Autodesk Fusion 360 part; units mm, degrees
note: some values were not read from the file. Set by a fixed rule: which sketch regions a step uses.
(part 4 of 20)
  spline S18 degree 5 poles (-22.7084, -21.1029) (-22.7059, -21.1018) (-22.7009, -21.0998) (-22.6934, -21.0967) (-22.6834, -21.0925) (-22.671, -21.0873) (-22.6586, -21.0822) (-22.6462, -21.077) (-22.6339, -21.0718) (-22.6217, -21.0666) (-22.6094, -21.0614) (-22.5972, -21.0562) (-22.585, -21.051) (-22.5729, -21.0458) (-22.5608, -21.0406) (-22.5487, -21.0354) (-22.5367, -21.0302) (-22.5247, -21.025) (-22.5127, -21.0198) (-22.5008, -21.0145) (-22.4889, -21.0093) (-22.4771, -21.0041) (-22.4653, -20.9989) (-22.4535, -20.9937) (-22.4417, -20.9884) (-22.43, -20.9832) (-22.4184, -20.978) (-22.4067, -20.9727) (-22.3951, -20.9675) (-22.3836, -20.9623) (-22.3721, -20.957) (-22.3606, -20.9518) (-22.3491, -20.9466) (-22.3377, -20.9413) (-22.3264, -20.9361) (-22.315, -20.9308) (-22.3037, -20.9256) (-22.2925, -20.9204) (-22.2812, -20.9151) (-22.2701, -20.9099) (-22.2589, -20.9046) (-22.2478, -20.8994) (-22.2367, -20.8942) (-22.2257, -20.8889) (-22.2147, -20.8837) (-22.2038, -20.8784) (-22.1928, -20.8732) (-22.182, -20.868) (-22.1711, -20.8627) (-22.1603, -20.8575) (-22.1496, -20.8523) (-22.1388, -20.847) (-22.1281, -20.8418) (-22.1175, -20.8366) (-22.1069, -20.8313) (-22.0963, -20.8261) (-22.0858, -20.8209) (-22.0753, -20.8157) (-22.0649, -20.8105) (-22.0544, -20.8052) (-22.0441, -20.8) (-22.0337, -20.7948) (-22.0235, -20.7896) (-22.0132, -20.7844) (-22.003, -20.7792) (-21.9928, -20.774) (-21.9827, -20.7688) (-21.9726, -20.7636) (-21.9625, -20.7584) (-21.9525, -20.7532) (-21.9426, -20.748) (-21.9326, -20.7429) (-21.9228, -20.7377) (-21.9129, -20.7325) (-21.9031, -20.7274) (-21.8933, -20.7222) (-21.8836, -20.717) (-21.8739, -20.7119) (-21.8643, -20.7067) (-21.8547, -20.7016) (-21.8451, -20.6965) (-21.8356, -20.6913) (-21.8261, -20.6862) (-21.8167, -20.6811) (-21.8073, -20.676) (-21.798, -20.6709) (-21.7887, -20.6658) (-21.7794, -20.6607) (-21.7702, -20.6556) (-21.761, -20.6505) (-21.7519, -20.6454) (-21.7428, -20.6404) (-21.7337, -20.6353) (-21.7247, -20.6303) (-21.7158, -20.6252) (-21.7068, -20.6202) (-21.698, -20.6152) (-21.6891, -20.6101) (-21.6803, -20.6051) (-21.6716, -20.6001) (-21.6629, -20.5951) (-21.6542, -20.5902) (-21.6456, -20.5852) (-21.6371, -20.5802) (-21.6285, -20.5753) (-21.6201, -20.5703) (-21.6116, -20.5654) (-21.6032, -20.5605) (-21.5949, -20.5555) (-21.5866, -20.5506) (-21.5783, -20.5457) (-21.5701, -20.5409) (-21.5619, -20.536) (-21.5538, -20.5311) (-21.5458, -20.5263) (-21.5377, -20.5214) (-21.5297, -20.5166) (-21.5218, -20.5118) (-21.5139, -20.507) (-21.5061, -20.5022) (-21.4983, -20.4974) (-21.4905, -20.4927) (-21.4828, -20.4879) (-21.4752, -20.4832) (-21.4676, -20.4784) (-21.46, -20.4737) (-21.4525, -20.469) (-21.445, -20.4644) (-21.4376, -20.4597) (-21.4302, -20.455) (-21.4229, -20.4504) (-21.4156, -20.4458) (-21.4084, -20.4412) (-21.4012, -20.4366) (-21.3941, -20.432) (-21.387, -20.4274) (-21.38, -20.4229) (-21.373, -20.4184) (-21.3661, -20.4139) (-21.3592, -20.4094) (-21.3523, -20.4049) (-21.3455, -20.4004) (-21.3388, -20.396) (-21.3321, -20.3916) (-21.3255, -20.3872) (-21.3189, -20.3828) (-21.3124, -20.3784) (-21.3059, -20.3741) (-21.2995, -20.3698) (-21.2931, -20.3655) (-21.2867, -20.3612) (-21.2805, -20.3569) (-21.2742, -20.3527) (-21.2681, -20.3484) (-21.2619, -20.3442) (-21.2559, -20.3401) (-21.2498, -20.3359) (-21.2439, -20.3318) (-21.238, -20.3277) (-21.2321, -20.3236) (-21.2263, -20.3195) (-21.2205, -20.3155) (-21.2148, -20.3115) (-21.2092, -20.3075) (-21.2036, -20.3035) (-21.1981, -20.2996) (-21.1926, -20.2956) (-21.1871, -20.2918) (-21.1818, -20.2879) (-21.1764, -20.2841) (-21.1712, -20.2802) (-21.166, -20.2765) (-21.1608, -20.2727) (-21.1557, -20.269) (-21.1507, -20.2653) (-21.1457, -20.2616) (-21.1408, -20.258) (-21.1359, -20.2544) (-21.1311, -20.2508) (-21.1263, -20.2472) (-21.1216, -20.2437) (-21.117, -20.2402) (-21.1124, -20.2368) (-21.1079, -20.2333) (-21.1034, -20.23) (-21.099, -20.2266) (-21.0947, -20.2233) (-21.0904, -20.22) (-21.0862, -20.2167) (-21.082, -20.2135) (-21.0779, -20.2103) (-21.0739, -20.2072) (-21.0699, -20.2041) (-21.066, -20.201) (-21.0621, -20.198) (-21.0583, -20.195) (-21.0546, -20.192) (-21.0509, -20.1891) (-21.0473, -20.1862) (-21.0437, -20.1834) (-21.0403, -20.1806) (-21.0368, -20.1778) (-21.0335, -20.1751) (-21.0302, -20.1724) (-21.027, -20.1698) (-21.0238, -20.1672) (-21.0207, -20.1647) (-21.0177, -20.1622) (-21.0148, -20.1597) (-21.0119, -20.1573) (-21.009, -20.155) (-21.0063, -20.1527) (-21.0036, -20.1504) (-21.001, -20.1482) (-20.9984, -20.1461) (-20.996, -20.144) (-20.9936, -20.1419) (-20.9912, -20.1399) (-20.989, -20.138) (-20.9868, -20.1361) (-20.9847, -20.1343) (-20.9826, -20.1325) (-20.9806, -20.1308) (-20.9787, -20.1291) (-20.9769, -20.1275) (-20.9752, -20.126) (-20.9735, -20.1245) (-20.9719, -20.123) (-20.9704, -20.1217) (-20.9689, -20.1204) (-20.9675, -20.1192) (-20.9663, -20.118) (-20.9651, -20.1169) (-20.9639, -20.1159) (-20.9629, -20.1149) (-20.9619, -20.114) (-20.961, -20.1132) (-20.9602, -20.1125) (-20.9595, -20.1118) (-20.9589, -20.1112) (-20.9583, -20.1107) (-20.958, -20.1104) (-20.9577, -20.1102) (-20.9576, -20.11) (-20.9575, -20.11) knots -1 -1 -1 -1 -1 -1 -0.99583333 -0.99166667 -0.9875 -0.98333333 -0.97916667 -0.975 -0.97083333 -0.96666667 -0.9625 -0.95833333 -0.95416667 -0.95 -0.94583333 -0.94166667 -0.9375 -0.93333333 -0.92916667 -0.925 -0.92083333 -0.91666667 -0.9125 -0.90833333 -0.90416667 -0.9 -0.89583333 -0.89166667 -0.8875 -0.88333333 -0.87916667 -0.875 -0.87083333 -0.86666667 -0.8625 -0.85833333 -0.85416667 -0.85 -0.84583333 -0.84166667 -0.8375 -0.83333333 -0.82916667 -0.825 -0.82083333 -0.81666667 -0.8125 -0.80833333 -0.80416667 -0.8 -0.79583333 -0.79166667 -0.7875 -0.78333333 -0.77916667 -0.775 -0.77083333 -0.76666667 -0.7625 -0.75833333 -0.75416667 -0.75 -0.74583333 -0.74166667 -0.7375 -0.73333333 -0.72916667 -0.725 -0.72083333 -0.71666667 -0.7125 -0.70833333 -0.70416667 -0.7 -0.69583333 -0.69166667 -0.6875 -0.68333333 -0.67916667 -0.675 -0.67083333 -0.66666667 -0.6625 -0.65833333 -0.65416667 -0.65 -0.64583333 -0.64166667 -0.6375 -0.63333333 -0.62916667 -0.625 -0.62083333 -0.61666667 -0.6125 -0.60833333 -0.60416667 -0.6 -0.59583333 -0.59166667 -0.5875 -0.58333333 -0.57916667 -0.575 -0.57083333 -0.56666667 -0.5625 -0.55833333 -0.55416667 -0.55 -0.54583333 -0.54166667 -0.5375 -0.53333333 -0.52916667 -0.525 -0.52083333 -0.51666667 -0.5125 -0.50833333 -0.50416667 -0.5 -0.49583333 -0.49166667 -0.4875 -0.48333333 -0.47916667 -0.475 -0.47083333 -0.46666667 -0.4625 -0.45833333 -0.45416667 -0.45 -0.44583333 -0.44166667 -0.4375 -0.43333333 -0.42916667 -0.425 -0.42083333 -0.41666667 -0.4125 -0.40833333 -0.40416667 -0.4 -0.39583333 -0.39166667 -0.3875 -0.38333333 -0.37916667 -0.375 -0.37083333 -0.36666667 -0.3625 -0.35833333 -0.35416667 -0.35 -0.34583333 -0.34166667 -0.3375 -0.33333333 -0.32916667 -0.325 -0.32083333 -0.31666667 -0.3125 -0.30833333 -0.30416667 -0.3 -0.29583333 -0.29166667 -0.2875 -0.28333333 -0.27916667 -0.275 -0.27083333 -0.26666667 -0.2625 -0.25833333 -0.25416667 -0.25 -0.24583333 -0.24166667 -0.2375 -0.23333333 -0.22916667 -0.225 -0.22083333 -0.21666667 -0.2125 -0.20833333 -0.20416667 -0.2 -0.19583333 -0.19166667 -0.1875 -0.18333333 -0.17916667 -0.175 -0.17083333 -0.16666667 -0.1625 -0.15833333 -0.15416667 -0.15 -0.14583333 -0.14166667 -0.1375 -0.13333333 -0.12916667 -0.125 -0.12083333 -0.11666667 -0.1125 -0.10833333 -0.10416667 -0.1 -0.09583333 -0.09166667 -0.0875 -0.08333333 -0.07916667 -0.075 -0.07083333 -0.06666667 -0.0625 -0.05833333 -0.05416667 -0.05 -0.04583333 -0.04166667 -0.0375 -0.03333333 -0.02916667 -0.025 -0.02083333 -0.01666667 -0.0125 -0.00833333 -0.00416667 0 0 0 0 0 0
  line L40 (-22.9448, -17.8091) -> (-22.9441, -17.8086)
  line L41 (-22.9441, -17.8086) -> (-22.7115, -17.6281)
  line L42 (-21.9649, -18.5501) -> (-22.1898, -18.7401)
  line L43 (-20.1094, -20.9569) -> (-20.11, -20.9575)
  line L44 (-19.9055, -20.7445) -> (-20.1094, -20.9569)
  line L45 (-26.6221, -10.8547) -> (-26.8948, -10.9659)
  line L46 (18.5501, -21.9649) -> (18.7401, -22.1898)
  line L47 (-27.3251, -9.8472) -> (-27.3243, -9.8469)
  line L48 (-22.1898, -18.7401) -> (-22.1904, -18.7406)
  arc A19 (-29.6298, -9.1146) -> (-29.3284, -10.0421) centre (0, 0) ccw
  line L49 (17.8091, -22.9448) -> (17.8086, -22.9441)
  spline S19 degree 5 poles (-24.7898, -18.6136) (-24.7872, -18.6128) (-24.782, -18.6113) (-24.7743, -18.609) (-24.7639, -18.6059) (-24.751, -18.6021) (-24.7382, -18.5982) (-24.7253, -18.5943) (-24.7125, -18.5905) (-24.6998, -18.5866) (-24.6871, -18.5827) (-24.6744, -18.5788) (-24.6617, -18.5749) (-24.6491, -18.571) (-24.6365, -18.5671) (-24.624, -18.5632) (-24.6115, -18.5593) (-24.599, -18.5553) (-24.5866, -18.5514) (-24.5742, -18.5475) (-24.5618, -18.5435) (-24.5495, -18.5395) (-24.5372, -18.5356) (-24.5249, -18.5316) (-24.5127, -18.5277) (-24.5005, -18.5237) (-24.4884, -18.5197) (-24.4762, -18.5157) (-24.4642, -18.5117) (-24.4521, -18.5077) (-24.4401, -18.5037) (-24.4281, -18.4997) (-24.4162, -18.4957) (-24.4043, -18.4917) (-24.3925, -18.4877) (-24.3806, -18.4836) (-24.3689, -18.4796) (-24.3571, -18.4756) (-24.3454, -18.4715) (-24.3337, -18.4675) (-24.3221, -18.4634) (-24.3105, -18.4594) (-24.299, -18.4553) (-24.2874, -18.4513) (-24.276, -18.4472) (-24.2645, -18.4431) (-24.2531, -18.4391) (-24.2417, -18.435) (-24.2304, -18.4309) (-24.2191, -18.4269) (-24.2079, -18.4228) (-24.1967, -18.4187) (-24.1855, -18.4146) (-24.1744, -18.4105) (-24.1633, -18.4064) (-24.1522, -18.4023) (-24.1412, -18.3982) (-24.1302, -18.3941) (-24.1193, -18.39) (-24.1084, -18.3859) (-24.0975, -18.3818) (-24.0867, -18.3777) (-24.0759, -18.3736) (-24.0652, -18.3695) (-24.0545, -18.3654) (-24.0438, -18.3613) (-24.0332, -18.3572) (-24.0226, -18.3531) (-24.0121, -18.349) (-24.0016, -18.3449) (-23.9911, -18.3408) (-23.9807, -18.3366) (-23.9703, -18.3325) (-23.96, -18.3284) (-23.9497, -18.3243) (-23.9395, -18.3202) (-23.9292, -18.3161) (-23.9191, -18.312) (-23.909, -18.3079) (-23.8989, -18.3038) (-23.8888, -18.2996) (-23.8788, -18.2955) (-23.8689, -18.2914) (-23.859, -18.2873) (-23.8491, -18.2832) (-23.8393, -18.2791) (-23.8295, -18.275) (-23.8197, -18.2709) (-23.81, -18.2668) (-23.8004, -18.2627) (-23.7907, -18.2587) (-23.7812, -18.2546) (-23.7716, -18.2505) (-23.7622, -18.2464) (-23.7527, -18.2423) (-23.7433, -18.2383) (-23.734, -18.2342) (-23.7247, -18.2301) (-23.7154, -18.226) (-23.7062, -18.222) (-23.697, -18.2179) (-23.6879, -18.2139) (-23.6788, -18.2098) (-23.6697, -18.2058) (-23.6607, -18.2018) (-23.6518, -18.1977) (-23.6429, -18.1937) (-23.634, -18.1897) (-23.6252, -18.1857) (-23.6165, -18.1816) (-23.6077, -18.1776) (-23.5991, -18.1736) (-23.5904, -18.1696) (-23.5818, -18.1657) (-23.5733, -18.1617) (-23.5648, -18.1577) (-23.5564, -18.1537) (-23.548, -18.1498) (-23.5396, -18.1458) (-23.5313, -18.1419) (-23.5231, -18.1379) (-23.5149, -18.134) (-23.5067, -18.1301) (-23.4986, -18.1262) (-23.4905, -18.1223) (-23.4825, -18.1184) (-23.4746, -18.1145) (-23.4666, -18.1106) (-23.4588, -18.1068) (-23.451, -18.1029) (-23.4432, -18.0991) (-23.4355, -18.0952) (-23.4278, -18.0914) (-23.4202, -18.0876) (-23.4126, -18.0838) (-23.4051, -18.08) (-23.3976, -18.0762) (-23.3902, -18.0724) (-23.3828, -18.0687) (-23.3755, -18.0649) (-23.3683, -18.0612) (-23.361, -18.0575) (-23.3539, -18.0538) (-23.3468, -18.0501) (-23.3397, -18.0464) (-23.3327, -18.0427) (-23.3257, -18.039) (-23.3188, -18.0354) (-23.312, -18.0318) (-23.3052, -18.0282) (-23.2984, -18.0246) (-23.2918, -18.021) (-23.2851, -18.0174) (-23.2785, -18.0139) (-23.272, -18.0103) (-23.2655, -18.0068) (-23.2591, -18.0033) (-23.2527, -17.9998) (-23.2464, -17.9963) (-23.2402, -17.9929) (-23.234, -17.9895) (-23.2278, -17.986) (-23.2217, -17.9826) (-23.2157, -17.9793) (-23.2097, -17.9759) (-23.2038, -17.9726) (-23.1979, -17.9692) (-23.1921, -17.9659) (-23.1864, -17.9627) (-23.1807, -17.9594) (-23.1751, -17.9562) (-23.1695, -17.9529) (-23.164, -17.9497) (-23.1585, -17.9466) (-23.1531, -17.9434) (-23.1478, -17.9403) (-23.1425, -17.9372) (-23.1373, -17.9341) (-23.1321, -17.931) (-23.127, -17.928) (-23.122, -17.925) (-23.117, -17.922) (-23.1121, -17.9191) (-23.1072, -17.9161) (-23.1024, -17.9132) (-23.0977, -17.9103) (-23.093, -17.9075) (-23.0884, -17.9047) (-23.0839, -17.9019) (-23.0794, -17.8991) (-23.075, -17.8964) (-23.0706, -17.8937) (-23.0664, -17.891) (-23.0621, -17.8883) (-23.058, -17.8857) (-23.0539, -17.8831) (-23.0499, -17.8806) (-23.0459, -17.8781) (-23.042, -17.8756) (-23.0382, -17.8731) (-23.0344, -17.8707) (-23.0308, -17.8683) (-23.0271, -17.866) (-23.0236, -17.8637) (-23.0201, -17.8614) (-23.0167, -17.8592) (-23.0134, -17.857) (-23.0101, -17.8548) (-23.0069, -17.8527) (-23.0038, -17.8506) (-23.0007, -17.8485) (-22.9978, -17.8465) (-22.9948, -17.8446) (-22.992, -17.8427) (-22.9893, -17.8408) (-22.9866, -17.8389) (-22.984, -17.8372) (-22.9814, -17.8354) (-22.979, -17.8337) (-22.9766, -17.8321) (-22.9743, -17.8305) (-22.9721, -17.8289) (-22.9699, -17.8274) (-22.9679, -17.826) (-22.9659, -17.8246) (-22.964, -17.8232) (-22.9622, -17.8219) (-22.9604, -17.8207) (-22.9588, -17.8195) (-22.9572, -17.8183) (-22.9557, -17.8172) (-22.9543, -17.8162) (-22.953, -17.8153) (-22.9518, -17.8144) (-22.9506, -17.8135) (-22.9496, -17.8127) (-22.9486, -17.812) (-22.9477, -17.8114) (-22.9469, -17.8108) (-22.9463, -17.8103) (-22.9457, -17.8098) (-22.9453, -17.8095) (-22.945, -17.8093) (-22.9448, -17.8092) (-22.9448, -17.8091) knots -1 -1 -1 -1 -1 -1 -0.99583333 -0.99166667 -0.9875 -0.98333333 -0.97916667 -0.975 -0.97083333 -0.96666667 -0.9625 -0.95833333 -0.95416667 -0.95 -0.94583333 -0.94166667 -0.9375 -0.93333333 -0.92916667 -0.925 -0.92083333 -0.91666667 -0.9125 -0.90833333 -0.90416667 -0.9 -0.89583333 -0.89166667 -0.8875 -0.88333333 -0.87916667 -0.875 -0.87083333 -0.86666667 -0.8625 -0.85833333 -0.85416667 -0.85 -0.84583333 -0.84166667 -0.8375 -0.83333333 -0.82916667 -0.825 -0.82083333 -0.81666667 -0.8125 -0.80833333 -0.80416667 -0.8 -0.79583333 -0.79166667 -0.7875 -0.78333333 -0.77916667 -0.775 -0.77083333 -0.76666667 -0.7625 -0.75833333 -0.75416667 -0.75 -0.74583333 -0.74166667 -0.7375 -0.73333333 -0.72916667 -0.725 -0.72083333 -0.71666667 -0.7125 -0.70833333 -0.70416667 -0.7 -0.69583333 -0.69166667 -0.6875 -0.68333333 -0.67916667 -0.675 -0.67083333 -0.66666667 -0.6625 -0.65833333 -0.65416667 -0.65 -0.64583333 -0.64166667 -0.6375 -0.63333333 -0.62916667 -0.625 -0.62083333 -0.61666667 -0.6125 -0.60833333 -0.60416667 -0.6 -0.59583333 -0.59166667 -0.5875 -0.58333333 -0.57916667 -0.575 -0.57083333 -0.56666667 -0.5625 -0.55833333 -0.55416667 -0.55 -0.54583333 -0.54166667 -0.5375 -0.53333333 -0.52916667 -0.525 -0.52083333 -0.51666667 -0.5125 -0.50833333 -0.50416667 -0.5 -0.49583333 -0.49166667 -0.4875 -0.48333333 -0.47916667 -0.475 -0.47083333 -0.46666667 -0.4625 -0.45833333 -0.45416667 -0.45 -0.44583333 -0.44166667 -0.4375 -0.43333333 -0.42916667 -0.425 -0.42083333 -0.41666667 -0.4125 -0.40833333 -0.40416667 -0.4 -0.39583333 -0.39166667 -0.3875 -0.38333333 -0.37916667 -0.375 -0.37083333 -0.36666667 -0.3625 -0.35833333 -0.35416667 -0.35 -0.34583333 -0.34166667 -0.3375 -0.33333333 -0.32916667 -0.325 -0.32083333 -0.31666667 -0.3125 -0.30833333 -0.30416667 -0.3 -0.29583333 -0.29166667 -0.2875 -0.28333333 -0.27916667 -0.275 -0.27083333 -0.26666667 -0.2625 -0.25833333 -0.25416667 -0.25 -0.24583333 -0.24166667 -0.2375 -0.23333333 -0.22916667 -0.225 -0.22083333 -0.21666667 -0.2125 -0.20833333 -0.20416667 -0.2 -0.19583333 -0.19166667 -0.1875 -0.18333333 -0.17916667 -0.175 -0.17083333 -0.16666667 -0.1625 -0.15833333 -0.15416667 -0.15 -0.14583333 -0.14166667 -0.1375 -0.13333333 -0.12916667 -0.125 -0.12083333 -0.11666667 -0.1125 -0.10833333 -0.10416667 -0.1 -0.09583333 -0.09166667 -0.0875 -0.08333333 -0.07916667 -0.075 -0.07083333 -0.06666667 -0.0625 -0.05833333 -0.05416667 -0.05 -0.04583333 -0.04166667 -0.0375 -0.03333333 -0.02916667 -0.025 -0.02083333 -0.01666667 -0.0125 -0.00833333 -0.00416667 0 0 0 0 0 0
  arc A20 (-21.1029, -22.7084) -> (-20.3781, -23.3609) centre (0, 0) ccw
  line L50 (22.9441, -17.8086) -> (22.9448, -17.8091)
  spline S20 degree 5 poles (-20.11, -20.9575) (-20.11, -20.9576) (-20.1102, -20.9577) (-20.1104, -20.958) (-20.1107, -20.9583) (-20.1112, -20.9589) (-20.1118, -20.9595) (-20.1125, -20.9602) (-20.1132, -20.961) (-20.114, -20.9619) (-20.1149, -20.9629) (-20.1159, -20.9639) (-20.1169, -20.9651) (-20.118, -20.9663) (-20.1192, -20.9675) (-20.1204, -20.9689) (-20.1217, -20.9704) (-20.123, -20.9719) (-20.1245, -20.9735) (-20.126, -20.9752) (-20.1275, -20.9769) (-20.1291, -20.9787) (-20.1308, -20.9806) (-20.1325, -20.9826) (-20.1343, -20.9847) (-20.1361, -20.9868) (-20.138, -20.989) (-20.1399, -20.9912) (-20.1419, -20.9936) (-20.144, -20.996) (-20.1461, -20.9984) (-20.1482, -21.001) (-20.1504, -21.0036) (-20.1527, -21.0063) (-20.155, -21.009) (-20.1573, -21.0119) (-20.1597, -21.0148) (-20.1622, -21.0177) (-20.1647, -21.0207) (-20.1672, -21.0238) (-20.1698, -21.027) (-20.1724, -21.0302) (-20.1751, -21.0335) (-20.1778, -21.0368) (-20.1806, -21.0403) (-20.1834, -21.0437) (-20.1862, -21.0473) (-20.1891, -21.0509) (-20.192, -21.0546) (-20.195, -21.0583) (-20.198, -21.0621) (-20.201, -21.066) (-20.2041, -21.0699) (-20.2072, -21.0739) (-20.2103, -21.0779) (-20.2135, -21.082) (-20.2167, -21.0862) (-20.22, -21.0904) (-20.2233, -21.0947) (-20.2266, -21.099) (-20.23, -21.1034) (-20.2333, -21.1079) (-20.2368, -21.1124) (-20.2402, -21.117) (-20.2437, -21.1216) (-20.2472, -21.1263) (-20.2508, -21.1311) (-20.2544, -21.1359) (-20.258, -21.1408) (-20.2616, -21.1457) (-20.2653, -21.1507) (-20.269, -21.1557) (-20.2727, -21.1608) (-20.2765, -21.166) (-20.2802, -21.1712) (-20.2841, -21.1764) (-20.2879, -21.1818) (-20.2918, -21.1871) (-20.2956, -21.1926) (-20.2996, -21.1981) (-20.3035, -21.2036) (-20.3075, -21.2092) (-20.3115, -21.2148) (-20.3155, -21.2205) (-20.3195, -21.2263) (-20.3236, -21.2321) (-20.3277, -21.238) (-20.3318, -21.2439) (-20.3359, -21.2498) (-20.3401, -21.2559) (-20.3442, -21.2619) (-20.3484, -21.2681) (-20.3527, -21.2742) (-20.3569, -21.2805) (-20.3612, -21.2867) (-20.3655, -21.2931) (-20.3698, -21.2995) (-20.3741, -21.3059) (-20.3784, -21.3124) (-20.3828, -21.3189) (-20.3872, -21.3255) (-20.3916, -21.3321) (-20.396, -21.3388) (-20.4004, -21.3455) (-20.4049, -21.3523) (-20.4094, -21.3592) (-20.4139, -21.3661) (-20.4184, -21.373) (-20.4229, -21.38) (-20.4274, -21.387) (-20.432, -21.3941) (-20.4366, -21.4012) (-20.4412, -21.4084) (-20.4458, -21.4156) (-20.4504, -21.4229) (-20.455, -21.4302) (-20.4597, -21.4376) (-20.4644, -21.445) (-20.469, -21.4525) (-20.4737, -21.46) (-20.4784, -21.4676) (-20.4832, -21.4752) (-20.4879, -21.4828) (-20.4927, -21.4905) (-20.4974, -21.4983) (-20.5022, -21.5061) (-20.507, -21.5139) (-20.5118, -21.5218) (-20.5166, -21.5297) (-20.5214, -21.5377) (-20.5263, -21.5458) (-20.5311, -21.5538) (-20.536, -21.5619) (-20.5409, -21.5701) (-20.5457, -21.5783) (-20.5506, -21.5866) (-20.5555, -21.5949) (-20.5605, -21.6032) (-20.5654, -21.6116) (-20.5703, -21.6201) (-20.5753, -21.6285) (-20.5802, -21.6371) (-20.5852, -21.6456) (-20.5902, -21.6542) (-20.5951, -21.6629) (-20.6001, -21.6716) (-20.6051, -21.6803) (-20.6101, -21.6891) (-20.6152, -21.698) (-20.6202, -21.7068) (-20.6252, -21.7158) (-20.6303, -21.7247) (-20.6353, -21.7337) (-20.6404, -21.7428) (-20.6454, -21.7519) (-20.6505, -21.761) (-20.6556, -21.7702) (-20.6607, -21.7794) (-20.6658, -21.7887) (-20.6709, -21.798) (-20.676, -21.8073) (-20.6811, -21.8167) (-20.6862, -21.8261) (-20.6913, -21.8356) (-20.6965, -21.8451) (-20.7016, -21.8547) (-20.7067, -21.8643) (-20.7119, -21.8739) (-20.717, -21.8836) (-20.7222, -21.8933) (-20.7274, -21.9031) (-20.7325, -21.9129) (-20.7377, -21.9228) (-20.7429, -21.9326) (-20.748, -21.9426) (-20.7532, -21.9525) (-20.7584, -21.9625) (-20.7636, -21.9726) (-20.7688, -21.9827) (-20.774, -21.9928) (-20.7792, -22.003) (-20.7844, -22.0132) (-20.7896, -22.0235) (-20.7948, -22.0337) (-20.8, -22.0441) (-20.8052, -22.0544) (-20.8105, -22.0649) (-20.8157, -22.0753) (-20.8209, -22.0858) (-20.8261, -22.0963) (-20.8313, -22.1069) (-20.8366, -22.1175) (-20.8418, -22.1281) (-20.847, -22.1388) (-20.8523, -22.1496) (-20.8575, -22.1603) (-20.8627, -22.1711) (-20.868, -22.182) (-20.8732, -22.1928) (-20.8784, -22.2038) (-20.8837, -22.2147) (-20.8889, -22.2257) (-20.8942, -22.2367) (-20.8994, -22.2478) (-20.9046, -22.2589) (-20.9099, -22.2701) (-20.9151, -22.2812) (-20.9204, -22.2925) (-20.9256, -22.3037) (-20.9308, -22.315) (-20.9361, -22.3264) (-20.9413, -22.3377) (-20.9466, -22.3491) (-20.9518, -22.3606) (-20.957, -22.3721) (-20.9623, -22.3836) (-20.9675, -22.3951) (-20.9727, -22.4067) (-20.978, -22.4184) (-20.9832, -22.43) (-20.9884, -22.4417) (-20.9937, -22.4535) (-20.9989, -22.4653) (-21.0041, -22.4771) (-21.0093, -22.4889) (-21.0145, -22.5008) (-21.0198, -22.5127) (-21.025, -22.5247) (-21.0302, -22.5367) (-21.0354, -22.5487) (-21.0406, -22.5608) (-21.0458, -22.5729) (-21.051, -22.585) (-21.0562, -22.5972) (-21.0614, -22.6094) (-21.0666, -22.6217) (-21.0718, -22.6339) (-21.077, -22.6462) (-21.0822, -22.6586) (-21.0873, -22.671) (-21.0925, -22.6834) (-21.0967, -22.6934) (-21.0998, -22.7009) (-21.1018, -22.7059) (-21.1029, -22.7084) knots 0 0 0 0 0 0 0.00416667 0.00833333 0.0125 0.01666667 0.02083333 0.025 0.02916667 0.03333333 0.0375 0.04166667 0.04583333 0.05 0.05416667 0.05833333 0.0625 0.06666667 0.07083333 0.075 0.07916667 0.08333333 0.0875 0.09166667 0.09583333 0.1 0.10416667 0.10833333 0.1125 0.11666667 0.12083333 0.125 0.12916667 0.13333333 0.1375 0.14166667 0.14583333 0.15 0.15416667 0.15833333 0.1625 0.16666667 0.17083333 0.175 0.17916667 0.18333333 0.1875 0.19166667 0.19583333 0.2 0.20416667 0.20833333 0.2125 0.21666667 0.22083333 0.225 0.22916667 0.23333333 0.2375 0.24166667 0.24583333 0.25 0.25416667 0.25833333 0.2625 0.26666667 0.27083333 0.275 0.27916667 0.28333333 0.2875 0.29166667 0.29583333 0.3 0.30416667 0.30833333 0.3125 0.31666667 0.32083333 0.325 0.32916667 0.33333333 0.3375 0.34166667 0.34583333 0.35 0.35416667 0.35833333 0.3625 0.36666667 0.37083333 0.375 0.37916667 0.38333333 0.3875 0.39166667 0.39583333 0.4 0.40416667 0.40833333 0.4125 0.41666667 0.42083333 0.425 0.42916667 0.43333333 0.4375 0.44166667 0.44583333 0.45 0.45416667 0.45833333 0.4625 0.46666667 0.47083333 0.475 0.47916667 0.48333333 0.4875 0.49166667 0.49583333 0.5 0.50416667 0.50833333 0.5125 0.51666667 0.52083333 0.525 0.52916667 0.53333333 0.5375 0.54166667 0.54583333 0.55 0.55416667 0.55833333 0.5625 0.56666667 0.57083333 0.575 0.57916667 0.58333333 0.5875 0.59166667 0.59583333 0.6 0.60416667 0.60833333 0.6125 0.61666667 0.62083333 0.625 0.62916667 0.63333333 0.6375 0.64166667 0.64583333 0.65 0.65416667 0.65833333 0.6625 0.66666667 0.67083333 0.675 0.67916667 0.68333333 0.6875 0.69166667 0.69583333 0.7 0.70416667 0.70833333 0.7125 0.71666667 0.72083333 0.725 0.72916667 0.73333333 0.7375 0.74166667 0.74583333 0.75 0.75416667 0.75833333 0.7625 0.76666667 0.77083333 0.775 0.77916667 0.78333333 0.7875 0.79166667 0.79583333 0.8 0.80416667 0.80833333 0.8125 0.81666667 0.82083333 0.825 0.82916667 0.83333333 0.8375 0.84166667 0.84583333 0.85 0.85416667 0.85833333 0.8625 0.86666667 0.87083333 0.875 0.87916667 0.88333333 0.8875 0.89166667 0.89583333 0.9 0.90416667 0.90833333 0.9125 0.91666667 0.92083333 0.925 0.92916667 0.93333333 0.9375 0.94166667 0.94583333 0.95 0.95416667 0.95833333 0.9625 0.96666667 0.97083333 0.975 0.97916667 0.98333333 0.9875 0.99166667 0.99583333 1 1 1 1 1 1
  line L51 (25.6019, -13.7175) -> (25.6012, -13.7171)
  spline S21 degree 5 poles (-26.8955, -10.9662) (-26.8956, -10.9662) (-26.8958, -10.9663) (-26.8961, -10.9664) (-26.8966, -10.9666) (-26.8973, -10.9669) (-26.8981, -10.9672) (-26.899, -10.9676) (-26.9, -10.9681) (-26.9011, -10.9685) (-26.9023, -10.9691) (-26.9036, -10.9696) (-26.905, -10.9702) (-26.9065, -10.9709) (-26.908, -10.9716) (-26.9097, -10.9724) (-26.9115, -10.9731) (-26.9134, -10.974) (-26.9153, -10.9749) (-26.9173, -10.9758) (-26.9195, -10.9768) (-26.9217, -10.9778) (-26.924, -10.9788) (-26.9263, -10.9799) (-26.9288, -10.9811) (-26.9313, -10.9823) (-26.9339, -10.9835) (-26.9366, -10.9848) (-26.9394, -10.9861) (-26.9423, -10.9875) (-26.9452, -10.9889) (-26.9482, -10.9903) (-26.9513, -10.9918) (-26.9544, -10.9934) (-26.9577, -10.9949) (-26.961, -10.9966) (-26.9643, -10.9982) (-26.9678, -10.9999) (-26.9713, -11.0017) (-26.9748, -11.0035) (-26.9785, -11.0053) (-26.9822, -11.0072) (-26.986, -11.0091) (-26.9898, -11.0111) (-26.9937, -11.0131) (-26.9977, -11.0151) (-27.0017, -11.0172) (-27.0058, -11.0193) (-27.01, -11.0215) (-27.0142, -11.0237) (-27.0185, -11.0259) (-27.0228, -11.0282) (-27.0272, -11.0306) (-27.0317, -11.0329) (-27.0362, -11.0353) (-27.0408, -11.0378) (-27.0454, -11.0403) (-27.0501, -11.0428) (-27.0549, -11.0454) (-27.0597, -11.048) (-27.0645, -11.0507) (-27.0694, -11.0534) (-27.0744, -11.0561) (-27.0794, -11.0589) (-27.0845, -11.0617) (-27.0896, -11.0646) (-27.0948, -11.0675) (-27.1, -11.0704) (-27.1053, -11.0734) (-27.1106, -11.0764) (-27.116, -11.0795) (-27.1214, -11.0826) (-27.1269, -11.0857) (-27.1324, -11.0889) (-27.138, -11.0921) (-27.1436, -11.0954) (-27.1493, -11.0987) (-27.155, -11.102) (-27.1608, -11.1054) (-27.1666, -11.1088) (-27.1725, -11.1123) (-27.1784, -11.1158) (-27.1843, -11.1193) (-27.1903, -11.1229) (-27.1963, -11.1265) (-27.2024, -11.1301) (-27.2085, -11.1338) (-27.2147, -11.1376) (-27.2209, -11.1413) (-27.2271, -11.1451) (-27.2334, -11.149) (-27.2397, -11.1529) (-27.2461, -11.1568) (-27.2525, -11.1608) (-27.259, -11.1648) (-27.2654, -11.1688) (-27.272, -11.1729) (-27.2785, -11.177) (-27.2851, -11.1812) (-27.2918, -11.1854) (-27.2985, -11.1896) (-27.3052, -11.1939) (-27.3119, -11.1982) (-27.3187, -11.2025) (-27.3256, -11.2069) (-27.3324, -11.2113) (-27.3393, -11.2158) (-27.3463, -11.2203) (-27.3533, -11.2248) (-27.3603, -11.2294) (-27.3673, -11.234) (-27.3744, -11.2387) (-27.3815, -11.2434) (-27.3887, -11.2481) (-27.3958, -11.2529) (-27.4031, -11.2577) (-27.4103, -11.2625) (-27.4176, -11.2674) (-27.4249, -11.2723) (-27.4323, -11.2773) (-27.4396, -11.2823) (-27.447, -11.2873) (-27.4545, -11.2924) (-27.462, -11.2975) (-27.4695, -11.3026) (-27.477, -11.3078) (-27.4846, -11.313) (-27.4922, -11.3183) (-27.4998, -11.3235) (-27.5074, -11.3289) (-27.5151, -11.3342) (-27.5228, -11.3396) (-27.5306, -11.3451) (-27.5384, -11.3506) (-27.5462, -11.3561) (-27.554, -11.3616) (-27.5618, -11.3672) (-27.5697, -11.3728) (-27.5776, -11.3785) (-27.5856, -11.3842) (-27.5936, -11.3899) (-27.6015, -11.3957) (-27.6096, -11.4015) (-27.6176, -11.4074) (-27.6257, -11.4132) (-27.6338, -11.4192) (-27.6419, -11.4251) (-27.6501, -11.4311) (-27.6582, -11.4371) (-27.6665, -11.4432) (-27.6747, -11.4493) (-27.6829, -11.4554) (-27.6912, -11.4616) (-27.6995, -11.4678) (-27.7078, -11.4741) (-27.7162, -11.4803) (-27.7246, -11.4867) (-27.733, -11.493) (-27.7414, -11.4994) (-27.7498, -11.5058) (-27.7583, -11.5123) (-27.7668, -11.5188) (-27.7753, -11.5253) (-27.7838, -11.5319) (-27.7924, -11.5385) (-27.801, -11.5452) (-27.8096, -11.5518) (-27.8182, -11.5585) (-27.8268, -11.5653) (-27.8355, -11.5721) (-27.8442, -11.5789) (-27.8529, -11.5858) (-27.8616, -11.5927) (-27.8704, -11.5996) (-27.8791, -11.6065) (-27.8879, -11.6135) (-27.8967, -11.6206) (-27.9055, -11.6276) (-27.9144, -11.6348) (-27.9233, -11.6419) (-27.9322, -11.6491) (-27.9411, -11.6563) (-27.95, -11.6635) (-27.9589, -11.6708) (-27.9679, -11.6781) (-27.9769, -11.6855) (-27.9859, -11.6929) (-27.9949, -11.7003) (-28.0039, -11.7078) (-28.013, -11.7153) (-28.0221, -11.7228) (-28.0312, -11.7303) (-28.0403, -11.7379) (-28.0494, -11.7456) (-28.0585, -11.7532) (-28.0677, -11.7609) (-28.0769, -11.7687) (-28.0861, -11.7765) (-28.0953, -11.7843) (-28.1045, -11.7921) (-28.1137, -11.8) (-28.123, -11.8079) (-28.1323, -11.8158) (-28.1416, -11.8238) (-28.1509, -11.8318) (-28.1602, -11.8399) (-28.1695, -11.848) (-28.1789, -11.8561) (-28.1882, -11.8643) (-28.1976, -11.8724) (-28.207, -11.8807) (-28.2164, -11.8889) (-28.2259, -11.8972) (-28.2353, -11.9055) (-28.2447, -11.9139) (-28.2542, -11.9223) (-28.2637, -11.9307) (-28.2732, -11.9392) (-28.2827, -11.9477) (-28.2922, -11.9562) (-28.3018, -11.9648) (-28.3113, -11.9734) (-28.3209, -11.982) (-28.3305, -11.9907) (-28.34, -11.9994) (-28.3496, -12.0081) (-28.3593, -12.0169) (-28.3689, -12.0257) (-28.3785, -12.0345) (-28.3882, -12.0434) (-28.3978, -12.0523) (-28.4075, -12.0613) (-28.4172, -12.0702) (-28.4269, -12.0792) (-28.4366, -12.0883) (-28.4464, -12.0973) (-28.4561, -12.1065) (-28.4658, -12.1156) (-28.4756, -12.1248) (-28.4854, -12.134) (-28.4951, -12.1432) (-28.503, -12.1506) (-28.5089, -12.1562) (-28.5128, -12.16) (-28.5147, -12.1618) knots 0 0 0 0 0 0 0.00416667 0.00833333 0.0125 0.01666667 0.02083333 0.025 0.02916667 0.03333333 0.0375 0.04166667 0.04583333 0.05 0.05416667 0.05833333 0.0625 0.06666667 0.07083333 0.075 0.07916667 0.08333333 0.0875 0.09166667 0.09583333 0.1 0.10416667 0.10833333 0.1125 0.11666667 0.12083333 0.125 0.12916667 0.13333333 0.1375 0.14166667 0.14583333 0.15 0.15416667 0.15833333 0.1625 0.16666667 0.17083333 0.175 0.17916667 0.18333333 0.1875 0.19166667 0.19583333 0.2 0.20416667 0.20833333 0.2125 0.21666667 0.22083333 0.225 0.22916667 0.23333333 0.2375 0.24166667 0.24583333 0.25 0.25416667 0.25833333 0.2625 0.26666667 0.27083333 0.275 0.27916667 0.28333333 0.2875 0.29166667 0.29583333 0.3 0.30416667 0.30833333 0.3125 0.31666667 0.32083333 0.325 0.32916667 0.33333333 0.3375 0.34166667 0.34583333 0.35 0.35416667 0.35833333 0.3625 0.36666667 0.37083333 0.375 0.37916667 0.38333333 0.3875 0.39166667 0.39583333 0.4 0.40416667 0.40833333 0.4125 0.41666667 0.42083333 0.425 0.42916667 0.43333333 0.4375 0.44166667 0.44583333 0.45 0.45416667 0.45833333 0.4625 0.46666667 0.47083333 0.475 0.47916667 0.48333333 0.4875 0.49166667 0.49583333 0.5 0.50416667 0.50833333 0.5125 0.51666667 0.52083333 0.525 0.52916667 0.53333333 0.5375 0.54166667 0.54583333 0.55 0.55416667 0.55833333 0.5625 0.56666667 0.57083333 0.575 0.57916667 0.58333333 0.5875 0.59166667 0.59583333 0.6 0.60416667 0.60833333 0.6125 0.61666667 0.62083333 0.625 0.62916667 0.63333333 0.6375 0.64166667 0.64583333 0.65 0.65416667 0.65833333 0.6625 0.66666667 0.67083333 0.675 0.67916667 0.68333333 0.6875 0.69166667 0.69583333 0.7 0.70416667 0.70833333 0.7125 0.71666667 0.72083333 0.725 0.72916667 0.73333333 0.7375 0.74166667 0.74583333 0.75 0.75416667 0.75833333 0.7625 0.76666667 0.77083333 0.775 0.77916667 0.78333333 0.7875 0.79166667 0.79583333 0.8 0.80416667 0.80833333 0.8125 0.81666667 0.82083333 0.825 0.82916667 0.83333333 0.8375 0.84166667 0.84583333 0.85 0.85416667 0.85833333 0.8625 0.86666667 0.87083333 0.875 0.87916667 0.88333333 0.8875 0.89166667 0.89583333 0.9 0.90416667 0.90833333 0.9125 0.91666667 0.92083333 0.925 0.92916667 0.93333333 0.9375 0.94166667 0.94583333 0.95 0.95416667 0.95833333 0.9625 0.96666667 0.97083333 0.975 0.97916667 0.98333333 0.9875 0.99166667 0.99583333 1 1 1 1 1 1
  arc A21 (20.3781, -23.3609) -> (21.1029, -22.7084) centre (0, 0) ccw
  spline S22 degree 5 poles (21.1029, -22.7084) (21.1018, -22.7059) (21.0998, -22.7009) (21.0967, -22.6934) (21.0925, -22.6834) (21.0873, -22.671) (21.0822, -22.6586) (21.077, -22.6462) (21.0718, -22.6339) (21.0666, -22.6217) (21.0614, -22.6094) (21.0562, -22.5972) (21.051, -22.585) (21.0458, -22.5729) (21.0406, -22.5608) (21.0354, -22.5487) (21.0302, -22.5367) (21.025, -22.5247) (21.0198, -22.5127) (21.0145, -22.5008) (21.0093, -22.4889) (21.0041, -22.4771) (20.9989, -22.4653) (20.9937, -22.4535) (20.9884, -22.4417) (20.9832, -22.43) (20.978, -22.4184) (20.9727, -22.4067) (20.9675, -22.3951) (20.9623, -22.3836) (20.957, -22.3721) (20.9518, -22.3606) (20.9466, -22.3491) (20.9413, -22.3377) (20.9361, -22.3264) (20.9308, -22.315) (20.9256, -22.3037) (20.9204, -22.2925) (20.9151, -22.2812) (20.9099, -22.2701) (20.9046, -22.2589) (20.8994, -22.2478) (20.8942, -22.2367) (20.8889, -22.2257) (20.8837, -22.2147) (20.8784, -22.2038) (20.8732, -22.1928) (20.868, -22.182) (20.8627, -22.1711) (20.8575, -22.1603) (20.8523, -22.1496) (20.847, -22.1388) (20.8418, -22.1281) (20.8366, -22.1175) (20.8313, -22.1069) (20.8261, -22.0963) (20.8209, -22.0858) (20.8157, -22.0753) (20.8105, -22.0649) (20.8052, -22.0544) (20.8, -22.0441) (20.7948, -22.0337) (20.7896, -22.0235) (20.7844, -22.0132) (20.7792, -22.003) (20.774, -21.9928) (20.7688, -21.9827) (20.7636, -21.9726) (20.7584, -21.9625) (20.7532, -21.9525) (20.748, -21.9426) (20.7429, -21.9326) (20.7377, -21.9228) (20.7325, -21.9129) (20.7274, -21.9031) (20.7222, -21.8933) (20.717, -21.8836) (20.7119, -21.8739) (20.7067, -21.8643) (20.7016, -21.8547) (20.6965, -21.8451) (20.6913, -21.8356) (20.6862, -21.8261) (20.6811, -21.8167) (20.676, -21.8073) (20.6709, -21.798) (20.6658, -21.7887) (20.6607, -21.7794) (20.6556, -21.7702) (20.6505, -21.761) (20.6454, -21.7519) (20.6404, -21.7428) (20.6353, -21.7337) (20.6303, -21.7247) (20.6252, -21.7158) (20.6202, -21.7068) (20.6152, -21.698) (20.6101, -21.6891) (20.6051, -21.6803) (20.6001, -21.6716) (20.5951, -21.6629) (20.5902, -21.6542) (20.5852, -21.6456) (20.5802, -21.6371) (20.5753, -21.6285) (20.5703, -21.6201) (20.5654, -21.6116) (20.5605, -21.6032) (20.5555, -21.5949) (20.5506, -21.5866) (20.5457, -21.5783) (20.5409, -21.5701) (20.536, -21.5619) (20.5311, -21.5538) (20.5263, -21.5458) (20.5214, -21.5377) (20.5166, -21.5297) (20.5118, -21.5218) (20.507, -21.5139) (20.5022, -21.5061) (20.4974, -21.4983) (20.4927, -21.4905) (20.4879, -21.4828) (20.4832, -21.4752) (20.4784, -21.4676) (20.4737, -21.46) (20.469, -21.4525) (20.4644, -21.445) (20.4597, -21.4376) (20.455, -21.4302) (20.4504, -21.4229) (20.4458, -21.4156) (20.4412, -21.4084) (20.4366, -21.4012) (20.432, -21.3941) (20.4274, -21.387) (20.4229, -21.38) (20.4184, -21.373) (20.4139, -21.3661) (20.4094, -21.3592) (20.4049, -21.3523) (20.4004, -21.3455) (20.396, -21.3388) (20.3916, -21.3321) (20.3872, -21.3255) (20.3828, -21.3189) (20.3784, -21.3124) (20.3741, -21.3059) (20.3698, -21.2995) (20.3655, -21.2931) (20.3612, -21.2867) (20.3569, -21.2805) (20.3527, -21.2742) (20.3484, -21.2681) (20.3442, -21.2619) (20.3401, -21.2559) (20.3359, -21.2498) (20.3318, -21.2439) (20.3277, -21.238) (20.3236, -21.2321) (20.3195, -21.2263) (20.3155, -21.2205) (20.3115, -21.2148) (20.3075, -21.2092) (20.3035, -21.2036) (20.2996, -21.1981) (20.2956, -21.1926) (20.2918, -21.1871) (20.2879, -21.1818) (20.2841, -21.1764) (20.2802, -21.1712) (20.2765, -21.166) (20.2727, -21.1608) (20.269, -21.1557) (20.2653, -21.1507) (20.2616, -21.1457) (20.258, -21.1408) (20.2544, -21.1359) (20.2508, -21.1311) (20.2472, -21.1263) (20.2437, -21.1216) (20.2402, -21.117) (20.2368, -21.1124) (20.2333, -21.1079) (20.23, -21.1034) (20.2266, -21.099) (20.2233, -21.0947) (20.22, -21.0904) (20.2167, -21.0862) (20.2135, -21.082) (20.2103, -21.0779) (20.2072, -21.0739) (20.2041, -21.0699) (20.201, -21.066) (20.198, -21.0621) (20.195, -21.0583) (20.192, -21.0546) (20.1891, -21.0509) (20.1862, -21.0473) (20.1834, -21.0437) (20.1806, -21.0403) (20.1778, -21.0368) (20.1751, -21.0335) (20.1724, -21.0302) (20.1698, -21.027) (20.1672, -21.0238) (20.1647, -21.0207) (20.1622, -21.0177) (20.1597, -21.0148) (20.1573, -21.0119) (20.155, -21.009) (20.1527, -21.0063) (20.1504, -21.0036) (20.1482, -21.001) (20.1461, -20.9984) (20.144, -20.996) (20.1419, -20.9936) (20.1399, -20.9912) (20.138, -20.989) (20.1361, -20.9868) (20.1343, -20.9847) (20.1325, -20.9826) (20.1308, -20.9806) (20.1291, -20.9787) (20.1275, -20.9769) (20.126, -20.9752) (20.1245, -20.9735) (20.123, -20.9719) (20.1217, -20.9704) (20.1204, -20.9689) (20.1192, -20.9675) (20.118, -20.9663) (20.1169, -20.9651) (20.1159, -20.9639) (20.1149, -20.9629) (20.114, -20.9619) (20.1132, -20.961) (20.1125, -20.9602) (20.1118, -20.9595) (20.1112, -20.9589) (20.1107, -20.9583) (20.1104, -20.958) (20.1102, -20.9577) (20.11, -20.9576) (20.11, -20.9575) knots -1 -1 -1 -1 -1 -1 -0.99583333 -0.99166667 -0.9875 -0.98333333 -0.97916667 -0.975 -0.97083333 -0.96666667 -0.9625 -0.95833333 -0.95416667 -0.95 -0.94583333 -0.94166667 -0.9375 -0.93333333 -0.92916667 -0.925 -0.92083333 -0.91666667 -0.9125 -0.90833333 -0.90416667 -0.9 -0.89583333 -0.89166667 -0.8875 -0.88333333 -0.87916667 -0.875 -0.87083333 -0.86666667 -0.8625 -0.85833333 -0.85416667 -0.85 -0.84583333 -0.84166667 -0.8375 -0.83333333 -0.82916667 -0.825 -0.82083333 -0.81666667 -0.8125 -0.80833333 -0.80416667 -0.8 -0.79583333 -0.79166667 -0.7875 -0.78333333 -0.77916667 -0.775 -0.77083333 -0.76666667 -0.7625 -0.75833333 -0.75416667 -0.75 -0.74583333 -0.74166667 -0.7375 -0.73333333 -0.72916667 -0.725 -0.72083333 -0.71666667 -0.7125 -0.70833333 -0.70416667 -0.7 -0.69583333 -0.69166667 -0.6875 -0.68333333 -0.67916667 -0.675 -0.67083333 -0.66666667 -0.6625 -0.65833333 -0.65416667 -0.65 -0.64583333 -0.64166667 -0.6375 -0.63333333 -0.62916667 -0.625 -0.62083333 -0.61666667 -0.6125 -0.60833333 -0.60416667 -0.6 -0.59583333 -0.59166667 -0.5875 -0.58333333 -0.57916667 -0.575 -0.57083333 -0.56666667 -0.5625 -0.55833333 -0.55416667 -0.55 -0.54583333 -0.54166667 -0.5375 -0.53333333 -0.52916667 -0.525 -0.52083333 -0.51666667 -0.5125 -0.50833333 -0.50416667 -0.5 -0.49583333 -0.49166667 -0.4875 -0.48333333 -0.47916667 -0.475 -0.47083333 -0.46666667 -0.4625 -0.45833333 -0.45416667 -0.45 -0.44583333 -0.44166667 -0.4375 -0.43333333 -0.42916667 -0.425 -0.42083333 -0.41666667 -0.4125 -0.40833333 -0.40416667 -0.4 -0.39583333 -0.39166667 -0.3875 -0.38333333 -0.37916667 -0.375 -0.37083333 -0.36666667 -0.3625 -0.35833333 -0.35416667 -0.35 -0.34583333 -0.34166667 -0.3375 -0.33333333 -0.32916667 -0.325 -0.32083333 -0.31666667 -0.3125 -0.30833333 -0.30416667 -0.3 -0.29583333 -0.29166667 -0.2875 -0.28333333 -0.27916667 -0.275 -0.27083333 -0.26666667 -0.2625 -0.25833333 -0.25416667 -0.25 -0.24583333 -0.24166667 -0.2375 -0.23333333 -0.22916667 -0.225 -0.22083333 -0.21666667 -0.2125 -0.20833333 -0.20416667 -0.2 -0.19583333 -0.19166667 -0.1875 -0.18333333 -0.17916667 -0.175 -0.17083333 -0.16666667 -0.1625 -0.15833333 -0.15416667 -0.15 -0.14583333 -0.14166667 -0.1375 -0.13333333 -0.12916667 -0.125 -0.12083333 -0.11666667 -0.1125 -0.10833333 -0.10416667 -0.1 -0.09583333 -0.09166667 -0.0875 -0.08333333 -0.07916667 -0.075 -0.07083333 -0.06666667 -0.0625 -0.05833333 -0.05416667 -0.05 -0.04583333 -0.04166667 -0.0375 -0.03333333 -0.02916667 -0.025 -0.02083333 -0.01666667 -0.0125 -0.00833333 -0.00416667 0 0 0 0 0 0
  line L52 (24.0278, -16.3184) -> (24.0271, -16.318)
  arc A22 (17.8246, -25.363) -> (18.6136, -24.7898) centre (0, 0) ccw
  spline S23 degree 5 poles (23.3609, -20.3781) (23.3596, -20.3757) (23.3571, -20.371) (23.3532, -20.3639) (23.348, -20.3544) (23.3416, -20.3426) (23.3351, -20.3308) (23.3287, -20.319) (23.3222, -20.3073) (23.3158, -20.2957) (23.3094, -20.284) (23.3029, -20.2724) (23.2965, -20.2609) (23.29, -20.2493) (23.2836, -20.2379) (23.2771, -20.2264) (23.2707, -20.215) (23.2643, -20.2036) (23.2578, -20.1922) (23.2514, -20.1809) (23.245, -20.1697) (23.2385, -20.1584) (23.2321, -20.1472) (23.2257, -20.136) (23.2193, -20.1249) (23.2128, -20.1138) (23.2064, -20.1028) (23.2, -20.0917) (23.1936, -20.0808) (23.1872, -20.0698) (23.1807, -20.0589) (23.1743, -20.048) (23.1679, -20.0372) (23.1615, -20.0264) (23.1551, -20.0156) (23.1487, -20.0049) (23.1423, -19.9942) (23.136, -19.9836) (23.1296, -19.973) (23.1232, -19.9624) (23.1168, -19.9518) (23.1104, -19.9413) (23.1041, -19.9309) (23.0977, -19.9205) (23.0914, -19.9101) (23.085, -19.8997) (23.0786, -19.8894) (23.0723, -19.8791) (23.066, -19.8689) (23.0596, -19.8587) (23.0533, -19.8486) (23.047, -19.8384) (23.0406, -19.8284) (23.0343, -19.8183) (23.028, -19.8083) (23.0217, -19.7984) (23.0154, -19.7884) (23.0091, -19.7785) (23.0029, -19.7687) (22.9966, -19.7589) (22.9903, -19.7491) (22.984, -19.7394) (22.9778, -19.7297) (22.9715, -19.72) (22.9653, -19.7104) (22.9591, -19.7009) (22.9528, -19.6913) (22.9466, -19.6818) (22.9404, -19.6724) (22.9342, -19.663) (22.928, -19.6536) (22.9218, -19.6443) (22.9156, -19.635) (22.9095, -19.6257) (22.9033, -19.6165) (22.8971, -19.6073) (22.891, -19.5982) (22.8849, -19.5891) (22.8787, -19.5801) (22.8726, -19.5711) (22.8665, -19.5621) (22.8604, -19.5532) (22.8543, -19.5443) (22.8483, -19.5354) (22.8422, -19.5266) (22.8361, -19.5179) (22.8301, -19.5091) (22.8241, -19.5005) (22.818, -19.4918) (22.812, -19.4832) (22.806, -19.4747) (22.8, -19.4662) (22.7941, -19.4577) (22.7881, -19.4493) (22.7822, -19.4409) (22.7762, -19.4325) (22.7703, -19.4242) (22.7644, -19.416) (22.7585, -19.4078) (22.7526, -19.3996) (22.7467, -19.3914) (22.7408, -19.3834) (22.735, -19.3753) (22.7292, -19.3673) (22.7233, -19.3593) (22.7175, -19.3514) (22.7118, -19.3436) (22.706, -19.3357) (22.7002, -19.3279) (22.6945, -19.3202) (22.6887, -19.3125) (22.683, -19.3048) (22.6773, -19.2972) (22.6716, -19.2897) (22.666, -19.2821) (22.6603, -19.2747) (22.6547, -19.2672) (22.6491, -19.2598) (22.6435, -19.2525) (22.6379, -19.2452) (22.6323, -19.2379) (22.6268, -19.2307) (22.6212, -19.2236) (22.6157, -19.2165) (22.6102, -19.2094) (22.6048, -19.2024) (22.5993, -19.1954) (22.5939, -19.1884) (22.5884, -19.1815) (22.583, -19.1747) (22.5777, -19.1679) (22.5723, -19.1611) (22.567, -19.1544) (22.5617, -19.1478) (22.5564, -19.1412) (22.5511, -19.1346) (22.5458, -19.1281) (22.5406, -19.1216) (22.5354, -19.1152) (22.5302, -19.1088) (22.525, -19.1025) (22.5199, -19.0962) (22.5148, -19.09) (22.5097, -19.0838) (22.5046, -19.0776) (22.4996, -19.0715) (22.4945, -19.0655) (22.4895, -19.0595) (22.4846, -19.0536) (22.4796, -19.0477) (22.4747, -19.0418) (22.4698, -19.036) (22.4649, -19.0303) (22.4601, -19.0246) (22.4553, -19.0189) (22.4505, -19.0133) (22.4457, -19.0077) (22.441, -19.0022) (22.4363, -18.9968) (22.4316, -18.9914) (22.427, -18.986) (22.4223, -18.9807) (22.4177, -18.9755) (22.4132, -18.9703) (22.4087, -18.9651) (22.4042, -18.96) (22.3997, -18.955) (22.3953, -18.95) (22.3909, -18.9451) (22.3865, -18.9402) (22.3821, -18.9353) (22.3778, -18.9306) (22.3736, -18.9258) (22.3693, -18.9211) (22.3651, -18.9165) (22.3609, -18.9119) (22.3568, -18.9074) (22.3527, -18.903) (22.3486, -18.8986) (22.3446, -18.8942) (22.3406, -18.8899) (22.3367, -18.8856) (22.3328, -18.8814) (22.3289, -18.8773) (22.325, -18.8732) (22.3212, -18.8692) (22.3175, -18.8652) (22.3138, -18.8613) (22.3101, -18.8574) (22.3065, -18.8536) (22.3029, -18.8499) (22.2993, -18.8462) (22.2958, -18.8426) (22.2923, -18.839) (22.2889, -18.8355) (22.2855, -18.832) (22.2822, -18.8286) (22.2789, -18.8252) (22.2757, -18.822) (22.2725, -18.8187) (22.2693, -18.8156) (22.2662, -18.8124) (22.2632, -18.8094) (22.2602, -18.8064) (22.2572, -18.8035) (22.2543, -18.8006) (22.2515, -18.7978) (22.2487, -18.7951) (22.2459, -18.7924) (22.2433, -18.7897) (22.2406, -18.7872) (22.238, -18.7847) (22.2355, -18.7823) (22.2331, -18.7799) (22.2307, -18.7776) (22.2283, -18.7753) (22.226, -18.7732) (22.2238, -18.771) (22.2216, -18.769) (22.2195, -18.767) (22.2175, -18.7651) (22.2155, -18.7632) (22.2136, -18.7615) (22.2117, -18.7597) (22.2099, -18.7581) (22.2082, -18.7565) (22.2066, -18.755) (22.205, -18.7536) (22.2035, -18.7522) (22.202, -18.7509) (22.2007, -18.7497) (22.1994, -18.7485) (22.1982, -18.7474) (22.197, -18.7464) (22.196, -18.7455) (22.195, -18.7446) (22.1941, -18.7438) (22.1933, -18.7431) (22.1925, -18.7424) (22.1919, -18.7419) (22.1913, -18.7414) (22.1909, -18.741) (22.1907, -18.7408) (22.1905, -18.7407) (22.1904, -18.7406) knots -1 -1 -1 -1 -1 -1 -0.99583333 -0.99166667 -0.9875 -0.98333333 -0.97916667 -0.975 -0.97083333 -0.96666667 -0.9625 -0.95833333 -0.95416667 -0.95 -0.94583333 -0.94166667 -0.9375 -0.93333333 -0.92916667 -0.925 -0.92083333 -0.91666667 -0.9125 -0.90833333 -0.90416667 -0.9 -0.89583333 -0.89166667 -0.8875 -0.88333333 -0.87916667 -0.875 -0.87083333 -0.86666667 -0.8625 -0.85833333 -0.85416667 -0.85 -0.84583333 -0.84166667 -0.8375 -0.83333333 -0.82916667 -0.825 -0.82083333 -0.81666667 -0.8125 -0.80833333 -0.80416667 -0.8 -0.79583333 -0.79166667 -0.7875 -0.78333333 -0.77916667 -0.775 -0.77083333 -0.76666667 -0.7625 -0.75833333 -0.75416667 -0.75 -0.74583333 -0.74166667 -0.7375 -0.73333333 -0.72916667 -0.725 -0.72083333 -0.71666667 -0.7125 -0.70833333 -0.70416667 -0.7 -0.69583333 -0.69166667 -0.6875 -0.68333333 -0.67916667 -0.675 -0.67083333 -0.66666667 -0.6625 -0.65833333 -0.65416667 -0.65 -0.64583333 -0.64166667 -0.6375 -0.63333333 -0.62916667 -0.625 -0.62083333 -0.61666667 -0.6125 -0.60833333 -0.60416667 -0.6 -0.59583333 -0.59166667 -0.5875 -0.58333333 -0.57916667 -0.575 -0.57083333 -0.56666667 -0.5625 -0.55833333 -0.55416667 -0.55 -0.54583333 -0.54166667 -0.5375 -0.53333333 -0.52916667 -0.525 -0.52083333 -0.51666667 -0.5125 -0.50833333 -0.50416667 -0.5 -0.49583333 -0.49166667 -0.4875 -0.48333333 -0.47916667 -0.475 -0.47083333 -0.46666667 -0.4625 -0.45833333 -0.45416667 -0.45 -0.44583333 -0.44166667 -0.4375 -0.43333333 -0.42916667 -0.425 -0.42083333 -0.41666667 -0.4125 -0.40833333 -0.40416667 -0.4 -0.39583333 -0.39166667 -0.3875 -0.38333333 -0.37916667 -0.375 -0.37083333 -0.36666667 -0.3625 -0.35833333 -0.35416667 -0.35 -0.34583333 -0.34166667 -0.3375 -0.33333333 -0.32916667 -0.325 -0.32083333 -0.31666667 -0.3125 -0.30833333 -0.30416667 -0.3 -0.29583333 -0.29166667 -0.2875 -0.28333333 -0.27916667 -0.275 -0.27083333 -0.26666667 -0.2625 -0.25833333 -0.25416667 -0.25 -0.24583333 -0.24166667 -0.2375 -0.23333333 -0.22916667 -0.225 -0.22083333 -0.21666667 -0.2125 -0.20833333 -0.20416667 -0.2 -0.19583333 -0.19166667 -0.1875 -0.18333333 -0.17916667 -0.175 -0.17083333 -0.16666667 -0.1625 -0.15833333 -0.15416667 -0.15 -0.14583333 -0.14166667 -0.1375 -0.13333333 -0.12916667 -0.125 -0.12083333 -0.11666667 -0.1125 -0.10833333 -0.10416667 -0.1 -0.09583333 -0.09166667 -0.0875 -0.08333333 -0.07916667 -0.075 -0.07083333 -0.06666667 -0.0625 -0.05833333 -0.05416667 -0.05 -0.04583333 -0.04166667 -0.0375 -0.03333333 -0.02916667 -0.025 -0.02083333 -0.01666667 -0.0125 -0.00833333 -0.00416667 0 0 0 0 0 0
  arc A23 (-27.0473, -9.7471) -> (-26.6221, -10.8547) centre (0, 0) ccw